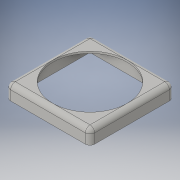
# Autodesk Inventor part: TrackDisplayTop
Saved by Autodesk Inventor 2016 (Build 200138000, 138)
## iProperties
Created: 2016-05-05
Part Number: TrackDisplayTop
Material: Generic
Document SubType Name: Modeling
Designer: xdlea
Density: 1 g/cm^3
Appearance: Default
Author: xdlea
Autodesk Inventor part; units mm, degrees
ref_plane "YZ Plane" through (0, 0, 0) normal (1, 0, 0) x (0, 1, 0)
ref_plane "XZ Plane" through (0, 0, 0) normal (0, 1, 0) x (-1, 0, 0)
ref_plane "XY Plane" through (0, 0, 0) normal (0, 0, 1) x (1, 0, 0)
sketch "Sketch1" plane through (0, 0, 0) normal (0, 1, 0) x (-1, 0, 0)
  circle A0 centre (0, 0) radius 25.4
  line L0 (-28.575, 28.575) -> (28.575, 28.575)
  line L1 (28.575, 28.575) -> (28.575, -28.575)
  line L2 (28.575, -28.575) -> (-28.575, -28.575)
  line L3 (-28.575, -28.575) -> (-28.575, 28.575)
  line L4 (-28.575, 28.575) -> (28.575, -28.575) construction
  line L5 (28.575, 28.575) -> (-28.575, -28.575) construction
  line L6 (-26.9875, 26.9875) -> (26.9875, 26.9875)
  line L7 (26.9875, 26.9875) -> (26.9875, -26.9875)
  line L8 (26.9875, -26.9875) -> (-26.9875, -26.9875)
  line L9 (-26.9875, -26.9875) -> (-26.9875, 26.9875)
  line L10 (-26.9875, 26.9875) -> (26.9875, -26.9875) construction
  line L11 (26.9875, 26.9875) -> (-26.9875, -26.9875) construction
  dimension "d0" = 50.8
  dimension "d2" = 28.575
  dimension "d7" = 26.9875
  constraints: 24 end point, 4 midpoint, 4 parallel, 4 perpendicular, 2 horizontal, 1 centre point, 1 coincident
  measures "d0" diameter of A0
  measures "d2" distance from line of L1 A0.centre
  measures "d7" distance from line of A0.centre L8
extrude "Extrusion1" add sketch "Sketch1" against normal blind 8.509 contours L0 L1 L2 L3
extrude "Extrusion2" add sketch "Sketch1" along normal blind 1.27 contours L0 L1 L2 L3 | L6 L7 L8 L9
fillet "Fillet1" radius 3.175 4 edges at (-28.575, -3.6195, -28.575) (28.575, -3.6195, -28.575) (28.575, -3.6195, 28.575) (-28.575, -3.6195, 28.575)
fillet "Fillet2" radius 3.175 8 edges at (27.6451, 1.27, -27.6451) (0, 1.27, -28.575) (-27.6451, 1.27, -27.6451) (-28.575, 1.27, 0) (-27.6451, 1.27, 27.6451) (0, 1.27, 28.575) (27.6451, 1.27, 27.6451) (28.575, 1.27, 0)
body "Solid1"
